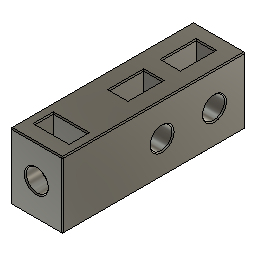
Hilfsanschlag Nutstein v3 (Autodesk Fusion 360 design; units mm, degrees)
Autodesk Fusion 360 part; units mm, degrees
sketch "Sketch1" plane through (0, 0, 0) normal (0, 1, 0) x (1, 0, 0)
  line L0 (0, 0) -> (20, 0)
  line L1 (20, 0) -> (20, -25.4)
  line L2 (20, -25.4) -> (0, -25.4)
  line L3 (0, -25.4) -> (0, 0)
  line L4 (10, -25.4) -> (10, 0) construction
  line L5 (16.5, -16.4528) -> (16.5, -8.9472)
  line L6 (16.5, -8.9472) -> (10, -5.1944)
  line L7 (10, -5.1944) -> (3.5, -8.9472)
  line L8 (3.5, -8.9472) -> (3.5, -16.4528)
  line L9 (3.5, -16.4528) -> (10, -20.2056)
  line L10 (10, -20.2056) -> (16.5, -16.4528)
  circle A0 centre (10, -12.7) radius 4.2
  line L11 (16.5, -16.4528) -> (16.5, -25.4)
  line L12 (3.5, -16.4528) -> (3.5, -25.4)
  point P0 (10, -12.7)
  dimension "d1" = 20
  dimension "d2" = 25.4
  dimension "d3" = 13
  dimension "d4" = 8.4
  constraint horizontal L0
  constraint vertical L1
  constraint horizontal L2
  constraint vertical L3
  constraint coincident L0.start L3.end
  constraint midpoint L2 L4.start
  constraint midpoint L0 L4.end
  constraint midpoint L4 P0
  constraint vertical L5
  constraint coincident P0 A0.centre
  constraint coincident L2 L11.end
  constraint perpendicular L2 L11
  constraint coincident L2 L12.end
  constraint perpendicular L2 L12
  measures "d1" distance of L1.end L2.end
  measures "d2" distance of L0.end L1.end
  measures "d3" distance of L5 L8
  measures "d4" diameter of A0
extrude "Extrude1" add sketch "Sketch1" along normal blind 70 contours L0 L1 L2 L3 L5 L6 L7 L8 L11 L12 | L2 L9 L10 L11 L12 | L5 L6 L7 L8 L9 L10 | A0
extrude "Extrude5" cut sketch "Sketch1" along normal blind 25 contours A0
extrude "Extrude2" cut sketch "Sketch1" along normal blind 7 from surface at 6 contours L2 L9 L10 L11 L12 | L5 L6 L7 L8 L9 L10
sketch "Sketch2" plane through (0, 0, 0) normal (-1, 0, 0) x (0, -1, 0)
  line L0 (0, 0) -> (0, 25.4)
  line L1 (0, 25.4) -> (-70, 25.4)
  line L2 (-70, 25.4) -> (-70, 0)
  line L3 (-70, 0) -> (0, 0)
  line L4 (-70, 12.7) -> (0, 12.7) construction
  line L5 (-58, 5.1944) -> (-51.5, 8.9472)
  line L6 (-51.5, 8.9472) -> (-51.5, 16.4528)
  line L7 (-51.5, 16.4528) -> (-58, 20.2056)
  line L8 (-58, 20.2056) -> (-64.5, 16.4528)
  line L9 (-64.5, 16.4528) -> (-64.5, 8.9472)
  line L10 (-64.5, 8.9472) -> (-58, 5.1944)
  circle A0 centre (-58, 12.7) radius 4.2
  line L11 (-64.5, 16.4528) -> (-64.5, 25.4)
  line L12 (-51.5, 16.4528) -> (-51.5, 25.4)
  circle A1 centre (-38, 12.7) radius 4.2
  line L13 (-31.5, 8.9472) -> (-31.5, 16.4528)
  line L14 (-31.5, 16.4528) -> (-38, 20.2056)
  line L15 (-38, 20.2056) -> (-44.5, 16.4528)
  line L16 (-44.5, 16.4528) -> (-44.5, 8.9472)
  line L17 (-44.5, 8.9472) -> (-38, 5.1944)
  line L18 (-38, 5.1944) -> (-31.5, 8.9472)
  line L19 (-44.5, 16.4528) -> (-44.5, 25.4)
  line L20 (-31.5, 16.4528) -> (-31.5, 25.4)
  point P0 (-58, 12.7)
  point P1 (-38, 12.7)
  dimension "d11" = 12
  dimension "d12" = 13
  dimension "d13" = 8.4
  dimension "d20" = 20
  constraint midpoint L2 L4.start
  constraint midpoint L0 L4.end
  constraint coincident L4 P0
  constraint vertical L6
  constraint coincident P0 A0.centre
  constraint coincident L1 L11.end
  constraint perpendicular L1 L11
  constraint coincident L1 L12.end
  constraint perpendicular L1 L12
  constraint coincident L4 P1
  constraint coincident P1 A1.centre
  constraint vertical L13
  constraint equal A0 A1
  constraint equal L7 L15
  constraint coincident L1 L19.end
  constraint perpendicular L1 L19
  constraint coincident L1 L20.end
  constraint perpendicular L1 L20
  measures "d11" distance of L4.start P0
  measures "d12" distance of L6 L9
  measures "d13" diameter of A0
  measures "d20" distance of P0 P1
extrude "Extrude3" cut sketch "Sketch2" against normal blind 24 contours A0 | A1
extrude "Extrude4" cut sketch "Sketch2" against normal blind 7 from surface at -6.5 contours L1 L14 L15 L19 L20 | L13 L14 L15 L16 L17 L18 | L1 L7 L8 L11 L12 | L5 L6 L7 L8 L9 L10
chamfer "Chamfer1" distance 0.4 angle 45 29 edges at (0, 70, 12.7) (20, 70, 12.7) (20, 0, 12.7) (0, 0, 12.7) (0, 35, 0) (0, 35, 25.4) (10, 0, 0) (10, 0, 25.4) (20, 35, 25.4) (10, 70, 25.4) (10, 64.5, 25.4) (6.5, 58, 25.4) (13.5, 58, 25.4) (10, 51.5, 25.4) (10, 13, 25.4) (16.5, 9.5, 25.4) (10, 6, 25.4) (3.5, 9.5, 25.4) (0, 61.9158, 14.2188) (10, 70, 0) (20, 61.9158, 11.1812) (20, 35, 0) (10, 44.5, 25.4) (13.5, 38, 25.4) (10, 31.5, 25.4) (6.5, 38, 25.4) (20, 41.9158, 11.1812) (6.0842, 0, 14.2188) (0, 41.9158, 14.2188)
